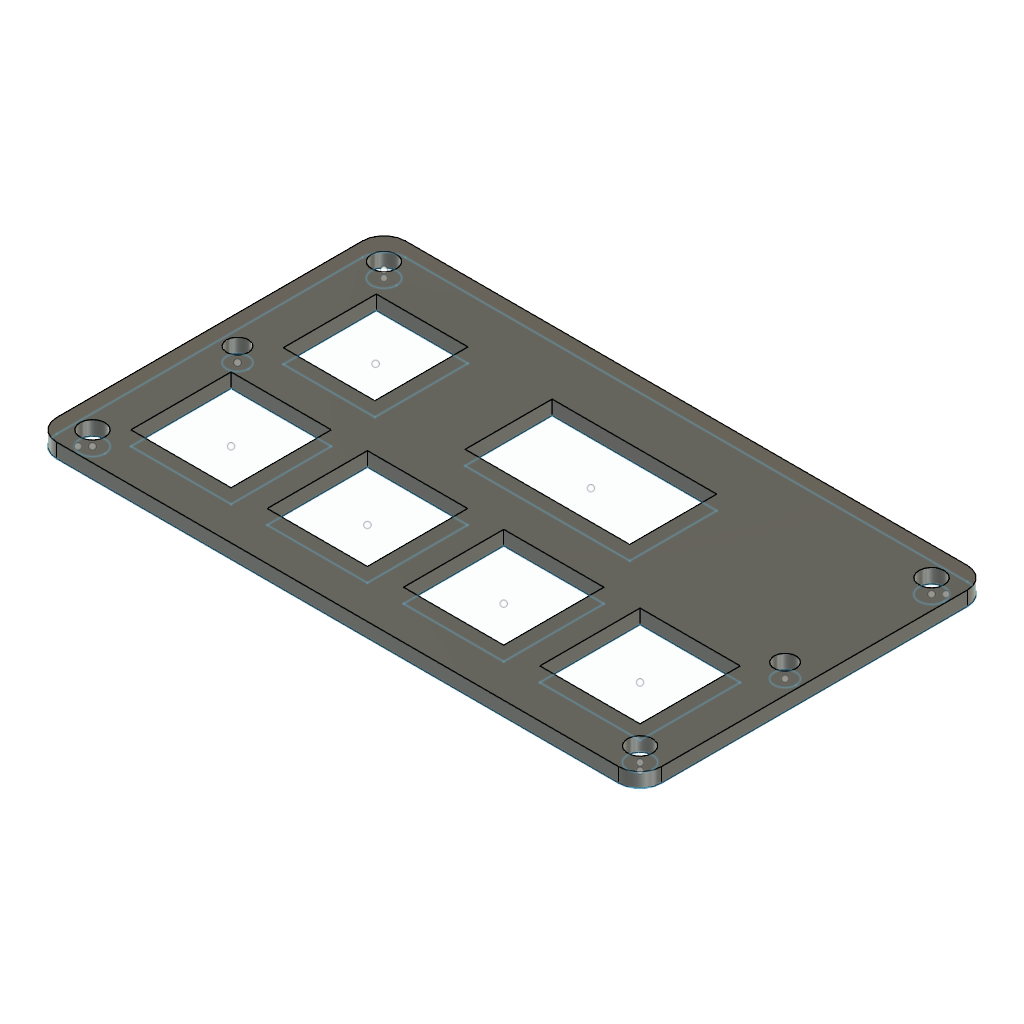
Hayai Top plate.f3d (Autodesk Fusion 360 design; units mm, degrees)
part number: 2026-09-20-15-53-54-702
Autodesk Fusion 360 part; units mm, degrees
sketch "Sketch1" plane through (0, 0, 0) normal (0, 0, 1) x (1, 0, 0)
  circle A0 centre (38.8472, 20.3675) radius 1.75
  circle A1 centre (38.8472, -0.0995) radius 1.525
  circle A2 centre (-37.6728, -20.3675) radius 1.75
  circle A3 centre (-37.6728, 20.3675) radius 1.75
  arc A4 (-38.6728, 24.3675) -> (-41.6728, 21.3675) centre (-38.6728, 21.3675) ccw
  line L0 (-38.6728, 24.3675) -> (39.8472, 24.3675)
  line L1 (-41.6728, -21.3675) -> (-41.6728, 21.3675)
  circle A5 centre (-37.6728, -0.0995) radius 1.525
  arc A6 (42.8472, 21.3675) -> (39.8472, 24.3675) centre (39.8472, 21.3675) ccw
  line L2 (42.8472, 21.3675) -> (42.8472, -21.3675)
  arc A7 (-41.6728, -21.3675) -> (-38.6728, -24.3675) centre (-38.6728, -21.3675) ccw
  line L3 (39.8472, -24.3675) -> (-38.6728, -24.3675)
  arc A8 (39.8472, -24.3675) -> (42.8472, -21.3675) centre (39.8472, -21.3675) ccw
  circle A9 centre (38.8472, -20.3675) radius 1.75
  line L4 (-20.9878, -3.6825) -> (-34.9878, -3.6825)
  line L5 (-34.9878, -3.6825) -> (-34.9878, -17.6825)
  line L6 (-34.9878, -17.6825) -> (-20.9878, -17.6825)
  line L7 (-20.9878, -17.6825) -> (-20.9878, -3.6825)
  line L8 (-1.9378, -17.6825) -> (-15.9378, -17.6825)
  line L9 (-15.9378, -17.6825) -> (-15.9378, -3.6825)
  line L10 (-15.9378, -3.6825) -> (-1.9378, -3.6825)
  line L11 (-1.9378, -3.6825) -> (-1.9378, -17.6825)
  line L12 (17.1122, -17.6825) -> (3.1122, -17.6825)
  line L13 (3.1122, -17.6825) -> (3.1122, -3.6825)
  line L14 (3.1122, -3.6825) -> (17.1122, -3.6825)
  line L15 (17.1122, -3.6825) -> (17.1122, -17.6825)
  line L16 (36.1622, -17.6825) -> (22.1622, -17.6825)
  line L17 (22.1622, -17.6825) -> (22.1622, -3.6825)
  line L18 (22.1622, -3.6825) -> (36.1622, -3.6825)
  line L19 (36.1622, -3.6825) -> (36.1622, -17.6825)
  line L20 (-21.4728, 2.8975) -> (-34.2728, 2.8975)
  line L21 (-34.2728, 2.8975) -> (-34.2728, 15.8975)
  line L22 (-34.2728, 15.8975) -> (-21.4728, 15.8975)
  line L23 (-21.4728, 15.8975) -> (-21.4728, 2.8975)
  line L24 (13.7272, 3.3125) -> (-9.2728, 3.3125)
  line L25 (-9.2728, 3.3125) -> (-9.2728, 15.4625)
  line L26 (-9.2728, 15.4625) -> (13.7272, 15.4625)
  line L27 (13.7272, 15.4625) -> (13.7272, 3.3125)
  point P0 (-27.9878, -10.6825)
  point P1 (-8.9378, -10.6825)
  point P2 (10.1122, -10.6825)
  point P3 (29.1622, -10.6825)
  point P4 (-27.8728, 9.3975)
  point P5 (2.2272, 9.3875)
  dimension "d44" = 3.05
  dimension "d45" = 3.05
  dimension "d46" = 20.268
  dimension "d47" = 3
  dimension "d48" = 3
  dimension "d49" = 3
  dimension "d50" = 3
  dimension "d51" = 3.5
  dimension "d52" = 4
  dimension "d53" = 1.4142
  dimension "d54" = 20.268
  dimension "d55" = 48.735
  dimension "d56" = 84.52
  dimension "d57" = 19.05
  dimension "d58" = 19.05
  dimension "d59" = 19.05
  dimension "d60" = 6.685
  dimension "d63" = 6.685
  dimension "d64" = 6.685
  dimension "d65" = 6.685
  dimension "d66" = 6.685
  dimension "d67" = 6.685
  dimension "d69" = 14
  dimension "d70" = 14
  dimension "d71" = 14
  dimension "d72" = 14
  dimension "d73" = 14
  dimension "d74" = 14
  dimension "d75" = 14
  dimension "d76" = 14
  dimension "d77" = 12.8
  dimension "d78" = 13
  dimension "d79" = 14.97
  dimension "d80" = 13.8
  dimension "d81" = 23
  dimension "d82" = 12.15
  dimension "d83" = 43.9
  dimension "d84" = 14.98
  dimension "d87" = 4
  dimension "d88" = 4
  dimension "d89" = 1.4142
  dimension "d92" = 4
  dimension "d93" = 1.4142
  dimension "d94" = 4
  dimension "d95" = 4
  constraint horizontal L0
  constraint vertical L2
  constraint horizontal L3
  constraint vertical L1
  constraint tangent A4 L0
  constraint tangent A4 L1
  constraint tangent L0 A6
  constraint tangent A6 L2
  constraint tangent L2 A8
  constraint tangent L3 A8
  constraint tangent A7 L3
  constraint tangent L1 A7
  constraint perpendicular L4 L5
  constraint parallel L4 L6
  constraint parallel L5 L7
  constraint perpendicular L8 L9
  constraint parallel L8 L10
  constraint parallel L9 L11
  constraint perpendicular L12 L13
  constraint parallel L12 L14
  constraint parallel L13 L15
  constraint perpendicular L16 L17
  constraint parallel L16 L18
  constraint parallel L17 L19
  constraint horizontal L20
  constraint perpendicular L20 L21
  constraint parallel L20 L22
  constraint parallel L21 L23
  constraint horizontal L24
  constraint perpendicular L24 L25
  constraint parallel L24 L26
  constraint parallel L25 L27
  constraint equal A0 A9
  constraint equal A0 A3
  constraint equal A2 A9
  measures "d44" diameter of A5
  measures "d45" diameter of A1
  measures "d46" distance of A5.centre A2.centre
  measures "d47" radius of A4
  measures "d48" radius of A6
  measures "d49" radius of A8
  measures "d50" radius of A7
  measures "d51" diameter of A9
  measures "d52" distance of L2 A9.centre
  measures "d53" distance of A8.centre A9.centre
  measures "d54" distance of A1.centre A9.centre
  measures "d55" distance of L0 L3
  measures "d56" distance of L1 L2
  measures "d57" distance of P0 P1
  measures "d58" distance of P1 P2
  measures "d59" distance of P2 P3
  measures "d60" distance of L2 L19
  measures "d63" distance of L1 L5
  measures "d64" distance of L3 L6
  measures "d65" distance of L3 L8
  measures "d66" distance of L3 L12
  measures "d67" distance of L3 L16
  measures "d69" distance of L4 L6
  measures "d70" distance of L5 L7
  measures "d71" distance of L9 L11
  measures "d72" distance of L8 L10
  measures "d73" distance of L12 L14
  measures "d74" distance of L13 L15
  measures "d75" distance of L16 L18
  measures "d76" distance of L17 L19
  measures "d77" distance of L21.end L22.end
  measures "d78" distance of L20.end L21.end
  measures "d79" distance of L0 P4
  measures "d80" distance of L1 P4
  measures "d81" distance of L25.end L26.end
  measures "d82" distance of L24.end L25.end
  measures "d83" distance of L1 P5
  measures "d84" distance of L0 P5
  measures "d87" distance of A3.centre L1
  measures "d88" distance of A0.centre L2
  measures "d89" distance of A0.centre A6.centre
  measures "d92" distance of A5.centre L1
  measures "d93" distance of A2.centre A7.centre
  measures "d94" distance of A2.centre L1
  measures "d95" distance of A1.centre L2
extrude "Extrude5" add sketch "Sketch1" along normal blind 2
extrude "Extrude1" [suppressed]
extrude "Extrude2" [suppressed]
extrude "Extrude3" [suppressed]
extrude "Extrude4" [suppressed]
equation "d53 = ( sqrt(2) ) * 1 mm"
equation "d89 = ( sqrt(2) ) * 1 mm"
